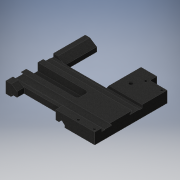
# Autodesk Inventor part: saddle
Saved by Autodesk Inventor 2016 (Build 200138000, 138)
## iProperties
Created: 2017-02-14
Part Number: saddle
Material: Iron, Cast
Document SubType Name: Modeling
Designer: M228544
Density: 7.15 g/cm^3
Appearance: Black Cast
Author: M228544
Autodesk Inventor part; units mm, degrees
ref_plane "YZ Plane" through (0, 0, 0) normal (1, 0, 0) x (0, 1, 0)
ref_plane "XZ Plane" through (0, 0, 0) normal (0, 1, 0) x (-1, 0, 0)
ref_plane "XY Plane" through (0, 0, 0) normal (0, 0, 1) x (1, 0, 0)
sketch "Sketch1" plane through (0, 0, 0) normal (0, 1, 0) x (-1, 0, 0)
  line L0 (0, 0) -> (-384, 0)
  line L1 (-384, 0) -> (-384, -343)
  line L2 (-384, -343) -> (0, -343)
  line L3 (0, -343) -> (0, 0)
  dimension "d0" = 384
  dimension "d1" = 343
  constraints: 8 end point, 2 parallel, 1 horizontal, 1 perpendicular
  measures "d0" distance of L2.end L1.end
  measures "d1" distance of L1.end L0.end
extrude "Extrusion1" add sketch "Sketch1" along normal blind 48.5
sketch "Sketch3" plane through (384, 0, 0) normal (1, 0, 0) x (0, 0, -1)
  line L0 (0, 0) -> (343, 0) projected
  line L1 (0, 0) -> (0, 48.5) projected
  line L2 (343, 0) -> (343, 48.5) projected
  line L3 (30, 48.5) -> (65, 48.5)
  line L4 (30, 48.5) -> (30, 37)
  line L5 (65, 48.5) -> (74.6496, 37)
  line L6 (43, 37) -> (74.6496, 37)
  line L7 (30, 37) -> (30, 35)
  line L8 (30, 35) -> (43, 35)
  line L9 (43, 35) -> (43, 37)
  dimension "d23" = 35
  dimension "d37" = 2
  dimension "d38" = 13
  constraints: 14 end point, 2 perpendicular, 1 horizontal, 1 vertical
  measures "d23" distance of L3.start L3.end
  measures "d37" distance of L4.end L7.end
  measures "d38" distance of L7.end L8.end
extrude "Extrusion2" cut sketch "Sketch3" against normal through all
sketch "Sketch7" plane through (384, 0, 0) normal (1, 0, 0) x (0, 0, -1)
  line L0 (65, 48.5) -> (343, 48.5) projected
  line L1 (65, 48.5) -> (161, 48.5)
  line L2 (161, 48.5) -> (174.2196, 48.5) construction
  line L3 (161, 48.5) -> (205, 48.5)
  line L4 (0, 0) -> (343, 0) projected
  line L5 (151.3504, 37) -> (192, 37)
  line L6 (205, 37) -> (205, 48.5)
  line L7 (161, 48.5) -> (151.3504, 37)
  line L8 (161, 48.5) -> (183.0653, 48.5) construction
  line L9 (205, 37) -> (205, 35)
  line L10 (205, 35) -> (192, 35)
  line L11 (192, 35) -> (192, 37)
  dimension "d27" = 96
  dimension "d29" = 44
  dimension "d32" = 130
  constraints: 20 end point, 3 horizontal, 3 perpendicular, 2 point on line, 1 vertical
  measures "d27" distance of L0.start L1.end
  measures "d29" distance of L1.end L3.end
  measures "d32" angle of L7 L8
extrude "Extrusion3" cut sketch "Sketch7" against normal through all
sketch "Sketch8" plane through (0, 48.5, 0) normal (0, 1, 0) x (1, 0, 0)
  line L0 (310, 343) -> (310, 316)
  line L1 (313, 313) -> (384, 313)
  line L2 (384, 0) -> (384, 343) projected
  line L3 (384, 313) -> (384, 343)
  line L4 (384, 343) -> (310, 343)
  line L5 (384, 343) -> (0, 343) projected
  arc A0 (310, 316) -> (313, 313) centre (313, 316) ccw
  point P0 (0, 0)
  point P1 (310, 313)
  dimension "d43" = 30
  dimension "d46" = 3
  constraints: 8 end point, 2 collinear, 2 point on circle, 2 point on line, 2 tangent, 1 centre point
  measures "d43" distance of L0.start point (310, 313)
  measures "d46" radius of A0
extrude "Extrusion4" cut sketch "Sketch8" against normal through all
sketch "Sketch12" plane through (0, 48.5, 0) normal (0, 1, 0) x (1, 0, 0)
  line L0 (221, 113) -> (221, 128)
  line L1 (211, 88) -> (0, 88)
  line L2 (211, 138) -> (0, 138)
  arc A0 (211, 88) -> (221, 98) centre (211, 98) ccw
  arc A1 (221, 128) -> (211, 138) centre (211, 128) ccw
  line L3 (221, 98) -> (221, 113)
  line L4 (0, 88) -> (0, 138)
  point P0 (384, 161)
  point P1 (221, 88)
  dimension "d72" = 10
  constraints: 10 end point, 4 point on circle, 3 tangent, 2 centre point, 2 point on line, 1 equal radius, 1 horizontal, 1 parallel, 1 perpendicular, 1 vertical
  measures "d72" radius of A0
extrude "Extrusion8" cut sketch "Sketch12" against normal blind 33
sketch "Sketch28" plane through (0, 48.5, 0) normal (0, 1, 0) x (1, 0, 0)
  circle A0 centre (373, 302) radius 5.8
  circle A1 centre (303.4, 302) radius 5.8
  circle A2 centre (373, 11) radius 5.8
  circle A3 centre (303.4, 11) radius 5.8
  point P0 (0, 0)
  point P1 (384, 313)
  point P2 (384, 0)
  dimension "d146" = 11.6
  dimension "d149" = 11.6
  dimension "d152" = 11.6
  dimension "d155" = 11.6
  constraints: 4 centre point
  measures "d146" diameter of A0
  measures "d149" diameter of A1
  measures "d152" diameter of A2
  measures "d155" diameter of A3
extrude "Extrusion19" cut sketch "Sketch28" against normal through all
sketch "Sketch29" plane through (0, 48.5, 0) normal (0, 0, 1) x (1, 0, 0)
  line L0 (0, -48.5) -> (0, 0) projected
  line L1 (0, 0) -> (384, 0) projected
  line L2 (23, 0) -> (48, -16.2352) projected
  line L3 (23, 0) -> (48, -16.2352)
  line L4 (0, -48.5) -> (384, -48.5) projected
  line L5 (23, 0) -> (48, 0)
  line L6 (48, -16.2352) -> (48, 0)
  line L7 (384, -13.5) -> (0, -13.5) projected
  point P0 (48, -48.5)
  point P1 (215, -48.5)
  point P2 (20, -48.5)
  constraints: 6 end point, 1 collinear, 1 perpendicular, 1 point on line
extrude "Extrusion20" cut sketch "Sketch29" against normal up to surface (30 mm away) contours L7 L6 L2 | L2 L1 L6 L7
sketch "Sketch30" plane through (0, 0, 0) normal (0, 0, 1) x (1, 0, 0)
  line L0 (48, 48.5) -> (215, 48.5)
  line L1 (215, 48.5) -> (215, 0)
  line L2 (215, 0) -> (48, 0)
  line L3 (48, 0) -> (48, 48.5)
  point P0 (0, 0)
  point P1 (48, 0)
  constraints: 8 end point, 2 parallel, 1 horizontal, 1 perpendicular
extrude "Extrusion21" cut sketch "Sketch30" against normal up to surface (30 mm away)
sketch "Sketch32" plane through (0, 48.5, 0) normal (0, 1, 0) x (1, 0, 0)
  line L0 (275, 266) -> (283, 266) construction
  circle A0 centre (280.6569, 260.3431) radius 8
  point P0 (0, 0)
  point P1 (255, 343)
  dimension "d168" = 16
  constraints: 2 end point, 1 centre point, 1 horizontal
  measures "d168" diameter of A0
extrude "Extrusion22" cut sketch "Sketch32" against normal blind 10
sketch "Sketch36" plane through (0, 0, -343) normal (0, 0, -1) x (-1, 0, 0)
  line L0 (-255, 0) -> (-243.6863, 11.3137)
  line L1 (-255, 0) -> (-239, 0) construction
  line L2 (-243.6863, 11.3137) -> (-239.0863, 11.3137)
  line L3 (-239.0863, 11.3137) -> (-229.7525, 1.9799)
  line L4 (-239.0863, 11.3137) -> (-225.8863, 11.3137) construction
  line L5 (-229.7525, 1.9799) -> (-217.7525, 1.9799)
  line L6 (-22, 0) -> (-22, 10)
  line L7 (-22, 10) -> (-55, 10)
  line L8 (-217.7525, 1.9799) -> (-217.7525, 0)
  line L9 (-55, 10) -> (-55, 0)
  line L10 (-255, 0) -> (-217.7525, 0)
  line L11 (-310, 0) -> (0, 0) projected
  line L12 (-55, 0) -> (-22, 0)
  dimension "d209" = 16
  dimension "d210" = 45
  dimension "d211" = 4.6
  dimension "d214" = 13.2
  dimension "d215" = 45
  dimension "d216" = 12
  dimension "d224" = 22
  dimension "d225" = 10
  constraints: 24 end point, 3 horizontal, 2 equal length, 2 perpendicular, 1 collinear, 1 vertical
  measures "d209" distance of L0.start L0.end
  measures "d210" angle of L1 L0
  measures "d211" distance of L0.end L2.end
  measures "d214" distance of L2.end L3.end
  measures "d215" angle of L3 L4
  measures "d216" distance of L3.end L5.end
  measures "d224" distance of L11.end L6.start
  measures "d225" distance of L6.start L6.end
extrude "Extrusion23" cut sketch "Sketch36" against normal through all
sketch "Sketch37" plane through (0, 0, -343) normal (0, 0, -1) x (-1, 0, 0)
  line L0 (-217.7525, 1.9799) -> (-217.7525, 15.9799)
  line L1 (-217.7525, 15.9799) -> (-241.3863, 48.5)
  line L2 (-241.3863, 48.5) -> (-19.5919, 48.5)
  line L3 (-211, 48.5) -> (0, 48.5) projected
  line L4 (-48, 10) -> (-55, 10) projected
  line L5 (-217.7525, 0) -> (-217.7525, 1.9799) projected
  line L6 (-217.7525, 1.9799) -> (-217.7525, 0)
  line L7 (-215, 0) -> (-55, 0) projected
  line L8 (-217.7525, 0) -> (-55, 0)
  line L9 (-55, 10) -> (-55, 0) projected
  line L10 (-55, 0) -> (-55, 10)
  line L11 (-217.7525, 15.9799) -> (-49.7525, 15.9799) construction
  line L12 (-55, 10) -> (-49.7525, 10)
  line L13 (-49.7525, 10) -> (-49.7525, 29)
  line L14 (-49.7525, 29) -> (-19.5919, 48.5)
  line L15 (0, 48.5) -> (-23, 48.5) projected
  point P0 (0, 0)
  dimension "d229" = 14
  dimension "d232" = 19
  constraints: 20 end point, 3 collinear, 2 point on line, 2 vertical, 1 horizontal, 1 perpendicular
  measures "d229" distance of L0.start L0.end
  measures "d232" distance of L12.end L13.end
extrude "Extrusion24" cut sketch "Sketch37" against normal blind 140
sketch "Sketch38" plane through (0, 0, -203) normal (0, 0, -1) x (-1, 0, 0)
  line L0 (-49.7525, 29) -> (-49.7525, 10) projected
  line L1 (-55, 9.9841) -> (-217.7525, 9.4921)
  line L2 (-217.7525, 1.9799) -> (-217.7525, 15.9799) projected
  line L3 (-217.7525, 0) -> (-217.7525, 1.9799) projected
  line L4 (-217.7525, 9.4921) -> (-217.7525, 0)
  line L5 (-215, 0) -> (-55, 0) projected
  line L6 (-217.7525, 0) -> (-55, 0)
  line L7 (-55, 10) -> (-55, 0) projected
  line L8 (-55, 0) -> (-55, 10)
  line L9 (-55, 10) -> (-55, 0)
  point P0 (0, 0)
  constraints: 10 end point, 2 collinear, 2 point on line, 1 perpendicular, 1 vertical
extrude "Extrusion25" cut sketch "Sketch38" against normal through all
sketch "Sketch40" plane through (0, 0, -343) normal (0, 0, -1) x (-1, 0, 0)
  line L0 (-229.5482, 9.4921) -> (-238.1559, 19.4995)
  line L1 (-229.5482, 9.4921) -> (-216.3482, 9.4921) construction
  line L2 (-238.1559, 19.4995) -> (-242.7559, 19.4995)
  line L3 (-242.7559, 19.4995) -> (-255, 9.1999)
  line L4 (-242.7559, 19.4995) -> (-226.7559, 19.4995) construction
  line L5 (-243.6863, 11.3137) -> (-255, 0) projected
  line L6 (-255, 9.1999) -> (-255, 0)
  line L7 (-229.5482, 9.4921) -> (-217.7525, 9.4921)
  line L8 (-217.7525, 9.4921) -> (-217.7525, 1.9799) projected
  line L9 (-217.7525, 9.4921) -> (-217.7525, 1.9799)
  line L10 (-217.7525, 1.9799) -> (-217.7525, 9.4921)
  line L11 (-217.7525, 1.9799) -> (-229.7525, 1.9799)
  line L12 (-229.7525, 1.9799) -> (-239.0863, 11.3137) projected
  line L13 (-229.7525, 1.9799) -> (-239.0863, 11.3137)
  line L14 (-239.0863, 11.3137) -> (-243.6863, 11.3137)
  line L15 (-255, 0) -> (-243.6863, 11.3137)
  dimension "d240" = 13.2
  dimension "d242" = 4.6
  dimension "d243" = 16
  constraints: 26 end point, 5 horizontal, 3 collinear, 2 equal length, 1 parallel, 1 perpendicular, 1 vertical
  measures "d240" distance of L0.start L0.end
  measures "d242" distance of L0.end L2.end
  measures "d243" distance of L2.end L3.end
extrude "Extrusion26" cut sketch "Sketch40" against normal through all
body "Solid1"
